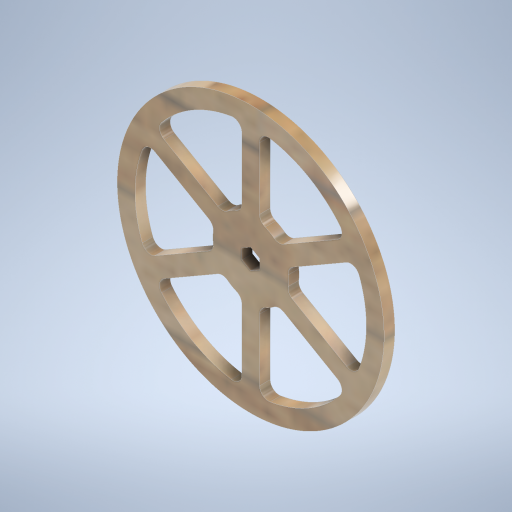
# Autodesk Inventor part: wheel
Saved by Autodesk Inventor 2023 (Build 270158000, 158)
## iProperties
Created: 2023-05-31
Part Number: wheel
Material: Hardboard
Document SubType Name: Sheet Metal
Designer: Ronan
Density: 0.799949 g/cm^3
Sheet Metal Rule: Default_mm
Appearance: Natural Maple - Glossy Dark Tint(1)
Mass: 41.1096 g
Surface Area: 253.901 cm^2
Volume: 51.3902 cm^3
Author: Ronan
Autodesk Inventor part; units mm, degrees
ref_plane "YZ Plane" through (0, 0, 0) normal (1, 0, 0) x (0, 1, 0)
ref_plane "XZ Plane" through (0, 0, 0) normal (0, 1, 0) x (-1, 0, 0)
ref_plane "XY Plane" through (0, 0, 0) normal (0, 0, 1) x (1, 0, 0)
sketch "Sketch1" plane through (0, 0, 0) normal (0, 0, 1) x (1, 0, 0)
  circle A0 centre (0, 0) radius 75
  line L0 (-90.1494, 78.9771) -> (78.0254, 78.9771) construction
  line L1 (78.0254, 78.9771) -> (78.0254, -87.6961) construction
  line L2 (78.0254, -87.6961) -> (-90.1494, -87.6961) construction
  line L3 (-90.1494, -87.6961) -> (-90.1494, 78.9771) construction
  line L4 (-5, 62.2697) -> (-5, 20.6534)
  line L5 (5, 20.6534) -> (5, 59.1608)
  line L6 (15.3864, 14.6568) -> (53.6249, 36.7338)
  line L7 (58.6249, 28.0736) -> (20.3864, 5.9966)
  line L8 (20.3864, -5.9966) -> (58.6249, -28.0736)
  line L9 (15.3864, -14.6568) -> (53.6249, -36.7338)
  line L10 (5, -20.6534) -> (5, -64.8074)
  line L11 (-5, -64.8074) -> (-5, -20.6534)
  line L12 (-15.3864, -14.6568) -> (-53.6249, -36.7338)
  line L13 (-58.6249, -28.0736) -> (-20.3864, -5.9966)
  line L14 (-20.3864, 5.9966) -> (-58.6249, 28.0736)
  line L15 (-53.6249, 36.7338) -> (-15.3864, 14.6568)
  line L16 (5, 59.1608) -> (5, 64.8074)
  line L17 (-5, 62.2697) -> (-5, 64.8074)
  arc A1 (10.8333, 64.0909) -> (5, 59.1608) centre (10, 59.1608) ccw
  arc A2 (-5, 64.8074) -> (-53.6249, 36.7338) centre (0, 0) ccw
  arc A3 (-5, 20.6534) -> (-15.3864, 14.6568) centre (0, 0) ccw
  arc A4 (15.3864, 14.6568) -> (5, 20.6534) centre (0, 0) ccw
  arc A5 (53.6249, 36.7338) -> (5, 64.8074) centre (0, 0) ccw
  arc A6 (58.6249, -28.0736) -> (58.6249, 28.0736) centre (0, 0) ccw
  arc A7 (20.3864, -5.9966) -> (20.3864, 5.9966) centre (0, 0) ccw
  arc A8 (5, -20.6534) -> (15.3864, -14.6568) centre (0, 0) ccw
  arc A9 (5, -64.8074) -> (53.6249, -36.7338) centre (0, 0) ccw
  arc A10 (-20.3864, 5.9966) -> (-20.3864, -5.9966) centre (0, 0) ccw
  arc A11 (-15.3864, -14.6568) -> (-5, -20.6534) centre (0, 0) ccw
  arc A12 (-58.6249, 28.0736) -> (-58.6249, -28.0736) centre (0, 0) ccw
  arc A13 (-53.6249, -36.7338) -> (-5, -64.8074) centre (0, 0) ccw
  line L18 (5, 2.8868) -> (5, -2.8868)
  line L19 (-5, 2.8868) -> (0, 5.7735)
  line L20 (5, 2.8868) -> (0, 5.7735)
  line L21 (-5, 2.8868) -> (-5, -2.8868)
  line L22 (0, -5.7735) -> (5, -2.8868)
  line L23 (-5, -2.8868) -> (0, -5.7735)
  line L24 (0, 0) -> (0, 5.7735)
  dimension "d5" = 150
  dimension "d41" = 10
  dimension "d54" = 5
  dimension "d74" = 120
  dimension "d76" = 120
  dimension "d77" = 120
  dimension "d78" = 120
  dimension "d79" = 120
  dimension "d80" = 120
  dimension "d81" = 10
  constraints: 42 end point, 27 point on circle, 14 centre point, 8 vertical, 4 coincident, 1 tangent, 2 other
  measures "d5" diameter of A0
  measures "d41" distance between parallel lines of L5 L4
  measures "d54" radius of A1
  measures "d74" angle of L22 L18
  measures "d76" angle of L23 L22
  measures "d77" angle of L23 L21
  measures "d78" angle of L21 L19
  measures "d79" angle of L19 L20
  measures "d80" angle of L20 L18
  measures "d81" distance between parallel lines of L18 L21
extrude "Extrusion1" add sketch "Sketch1" along normal blind 6
fillet "Fillet1" radius 5 1 edges at (5, 64.8074, 3)
fillet "Fillet2" radius 5 23 edges at (-53.6249, 36.7338, 3) (5, 20.6534, 3) (-53.6249, -36.7338, 3) (-58.6249, -28.0736, 3) (5, -64.8074, 3) (20.3864, -5.9966, 3) (15.3864, 14.6568, 3) (20.3864, 5.9966, 3) (15.3864, -14.6568, 3) (5, -20.6534, 3) (-20.3864, 5.9966, 3) (-15.3864, -14.6568, 3) (-5, -20.6534, 3) (53.6249, -36.7338, 3) (58.6249, 28.0736, 3) (-5, 64.8074, 3) (-5, 20.6534, 3) (-15.3864, 14.6568, 3) (58.6249, -28.0736, 3) (53.6249, 36.7338, 3) (-5, -64.8074, 3) (-20.3864, -5.9966, 3) (-58.6249, 28.0736, 3)
equation "\"BendRadius\" = Thickness"
equation "\"BendReliefWidth\" = Thickness"
equation "\"BendReliefDepth\" = 0.5 * Thickness"
equation "\"CornerReliefSize\" = 4 * Thickness"
equation "\"MinimumRemnant\" = 2 * Thickness"
equation "\"TransitionRadius\" = BendRadius"
equation "\"JacobiRadiusSize\" = BendRadius"
equation "\"GapSize\" = Thickness"
equation "\"Thickness\" = 0.5"
body "Solid1"
